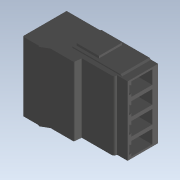
# Autodesk Inventor part: 5065752 4GD-1RR7.62-CLP-CBL
Saved by Autodesk Inventor 2021 (Build 250183000, 183)
## iProperties
Part Number: 5065752 4GD-1RR7.62-CLP-CBL
Material: Generic
Catalog Web Link: www.cadenas.de
Description: NEKM-C6 (p)-Terminal strip
Vendor: FESTO
Document SubType Name: Modeling
Designer: partserver
Manufacturer: FESTO
Mass: 15.9531 g
Surface Area: 83.8329 cm^2
Volume: 15.9531 cm^3
Density: 1 g/cm^3
Appearance: PSOLRGB-80-80-80
Categories: <MemberInstance><Categories><Category DisplayName="" Mnemonic="CABLEANDHARNESS" InternalName="e4a7e005-5e42-4d16-b293-125e7f0d0512"><Category DisplayName="" Mnemonic="CONNECTORS" InternalName="6f634eba-a678-4820-a31d-2c2d5ee6728e"><CategoryParameter DisplayName="" Mnemonic="REFDES" InternalName="c3740e8c-60ab-4d5d-8584-52b73222f2f0"/><Category DisplayName="" Mnemonic="DISCRETEWIRE" InternalName="9a3407de-09b2-4cdb-8c40-9708d5144a28"/></Category></Category></Categories><FamilyTemplate><FamilyTemplateParameters></FamilyTemplateParameters></FamilyTemplate><CategoryParameterMap><ParamToTemplateMap><ParamToTemplate CategoryParameter="//CategoryParameter[@InternalName='c3740e8c-60ab-4d5d-8584-52b73222f2f0']" ConstantValue=""/></ParamToTemplateMap></CategoryParameterMap></MemberInstance>
Category: PARTsolutions
Company: FESTO
PSOL_IDENT_0: {$CADENAS_DATA\23d-libs\festo\parts\n\nekm\parts\nekm_c6_parts.prj},199 {VTYP=3D},{NB=5065752 4GD-1R
PSOL_IDENT_1: R7.62-CLP-CBL},{LINA=5065752 4GD-1RR7.62-CLP-CBL},{NN=NEKM-C6 (p)},{DATE=16.05.2019 05:36:58},{GEOMD
PSOL_IDENT_2: ATE=16.05.2019 05:36:56},{VERSION=},{LINEID=80},{WBVAR=},{WBNUMERIC=}  {NB=5065752 4GD-1RR7.62-CLP-C
PSOL_IDENT_3: BL},{LINA=5065752 4GD-1RR7.62-CLP-CBL},{KT=DUMMY},{TNR=5065752},{TYP=4GD-1RR7.62-CLP-CBL},{VERS=5},{
PSOL_IDENT_4: N=4},{L=30.480},{L1=0.000}
NB: 5065752 4GD-1RR7.62-CLP-CBL
NN: NEKM-C6 (p)
NT: Terminal strip
NBSYN: $TNR. $TYP.
LINA: 5065752 4GD-1RR7.62-CLP-CBL
CATALOG: Festo
TNR: 5065752
TYP: 4GD-1RR7.62-CLP-CBL
VERS: 5
N: 4
L: 30.48
L1: 0
SUPPLIER: FESTO
ARTICLENO: 5065752 4GD-1RR7.62-CLP-CBL
BOMINFO: 5065752 4GD-1RR7.62-CLP-CBL
CREATOR: CADENAS GmbH
Title: 5065752 4GD-1RR7.62-CLP-CBL
Author: Cadenas PARTsolutions
Comments: Terminal strip
Autodesk Inventor part; units mm, degrees
sketch "Sketch_1" plane through (0, 0, 0) normal (0, 0, 1) x (1, 0, 0)
  line L0 (-14.7, -3.6) -> (-10.2, -3.6)
  arc A0 (-10, -3.8) -> (-10.2, -3.6) centre (-10.2, -3.8) ccw
  arc A1 (-10, -3.8) -> (-8.9, -4.9) centre (-8.9, -3.8) ccw
  line L1 (-8.9, -4.9) -> (4.3068, -4.9)
  line L2 (4.3068, -4.9) -> (4.5468, -7.6436)
  arc A2 (4.5468, -7.6436) -> (5.0449, -8.1) centre (5.0449, -7.6) ccw
  line L3 (5.0449, -8.1) -> (14.9, -8.1)
  line L4 (14.9, -8.1) -> (18.0177, -9.9)
  line L5 (18.0177, -9.9) -> (18.3, -9.9)
  arc A3 (18.3, -9.9) -> (18.5, -9.7) centre (18.3, -9.7) ccw
  line L6 (18.5, -9.7) -> (18.5, -9.6)
  line L7 (18.5, -9.6) -> (25.3, -9.6)
  arc A4 (25.3, -9.6) -> (25.8, -9.1) centre (25.3, -9.1) ccw
  line L8 (25.8, -9.1) -> (25.8, 9.9)
  line L9 (25.8, 9.9) -> (-14.7, 9.9)
  line L10 (-14.7, 9.9) -> (-14.7, -3.6)
  constraints: 22 end point, 10 point on circle, 5 centre point
extrude "Extrusion1" add sketch "Sketch_1" along normal mid plane 30.48
sketch "Sketch_2" plane through (0, 9.9, 0) normal (0, 1, 0) x (1, 0, 0)
  line L0 (-11.6, 15.24) -> (-11.6, -15.24)
  line L1 (-11.6, -15.24) -> (-10.8206, -15.69)
  line L2 (-10.8206, -15.69) -> (10.45, -15.69)
  line L3 (10.45, -15.69) -> (10.45, 15.69)
  line L4 (10.45, 15.69) -> (-10.8206, 15.69)
  line L5 (-10.8206, 15.69) -> (-11.6, 15.24)
  constraints: 12 end point
extrude "Extrusion2" add sketch "Sketch_2" against normal blind 12.825
sketch "Sketch_3" plane through (0, 0, 0) normal (0, 0, 1) x (1, 0, 0)
  line L0 (0, -1.625) -> (9.8, -1.625)
  line L1 (9.8, -1.625) -> (9.8, 8.575)
  line L2 (9.8, 8.575) -> (0, 8.575)
  line L3 (0, 8.575) -> (0, -1.625)
  constraints: 8 end point
extrude "Extrusion3" add sketch "Sketch_3" along normal mid plane 33.28
sketch "Sketch_4" plane through (26.75, 0, 0) normal (1, 0, 0) x (0, 0, -1)
  line L0 (-14.64, 6.0143) -> (-14.64, 3.1857)
  arc A0 (-14.64, 3.1857) -> (-8.22, 3.1857) centre (-11.43, 4.45) ccw
  line L1 (-8.22, 3.1857) -> (-8.22, 6.0143)
  arc A1 (-8.22, 6.0143) -> (-14.64, 6.0143) centre (-11.43, 4.75) ccw
  constraints: 4 end point, 4 point on circle, 2 centre point
extrude "Extrusion4" cut sketch "Sketch_4" against normal blind 10
pattern_linear "Rectangular Pattern1" count 4 spacing 7.62 along (0, 0, -1) of "Extrusion4"
sketch "Sketch_6" plane through (26.75, 0, 0) normal (1, 0, 0) x (0, 0, -1)
  line L0 (-13.28, -4.05) -> (-9.58, -4.05)
  line L1 (-9.58, -4.05) -> (-9.58, -0.2)
  line L2 (-9.58, -0.2) -> (-13.28, -0.2)
  line L3 (-13.28, -0.2) -> (-13.28, -4.05)
  constraints: 8 end point
extrude "Extrusion5" cut sketch "Sketch_6" against normal blind 7
pattern_linear "Rectangular Pattern2" count 4 spacing 7.62 along (0, 0, -1) of "Extrusion5"
sketch "Sketch_8" plane through (-14.7, 0, 0) normal (1, 0, 0) x (0, 0, -1)
  line L0 (-14.41, -1.925) -> (-13.1415, -1.925)
  arc A0 (-12.9485, -2.1178) -> (-13.1415, -1.925) centre (-13.1415, -2.118) ccw
  arc A1 (-13.0174, -2.2655) -> (-12.9485, -2.1178) centre (-13.1415, -2.1177) ccw
  line L1 (-13.0174, -2.2655) -> (-13.302, -2.5043)
  arc A2 (-13.302, -2.5043) -> (-13.1776, -2.846) centre (-13.1776, -2.6525) ccw
  line L2 (-13.1776, -2.846) -> (-9.6824, -2.846)
  arc A3 (-9.6824, -2.846) -> (-9.558, -2.5043) centre (-9.6824, -2.6525) ccw
  line L3 (-9.558, -2.5043) -> (-9.8426, -2.2655)
  arc A4 (-9.9115, -2.1178) -> (-9.8426, -2.2655) centre (-9.7185, -2.1177) ccw
  arc A5 (-9.7185, -1.925) -> (-9.9115, -2.1178) centre (-9.7185, -2.118) ccw
  line L4 (-9.7185, -1.925) -> (-8.45, -1.925)
  line L5 (-8.45, -1.925) -> (-8.45, 7.325)
  line L6 (-8.45, 7.325) -> (-14.41, 7.325)
  line L7 (-14.41, 7.325) -> (-14.41, -1.925)
  constraints: 16 end point, 12 point on circle, 6 centre point
extrude "Extrusion6" cut sketch "Sketch_8" along normal blind 14.7
pattern_linear "Rectangular Pattern3" count 4 spacing 7.62 along (0, 0, -1) of "Extrusion6"
sketch "Sketch_10" plane through (0, 0, 0) normal (1, 0, 0) x (0, 1, 0)
  circle A0 centre (3.475, 11.43) radius 1.6
  constraints: 1 centre point
extrude "Extrusion7" add sketch "Sketch_10" against normal blind 1
pattern_linear "Rectangular Pattern4" count 4 spacing 7.62 along (0, 0, -1) of "Extrusion7"
sketch "Sketch_12" plane through (0, 0, 0) normal (1, 0, 0) x (0, 1, 0)
  line L0 (3.075, 12.93) -> (3.075, 9.93)
  line L1 (3.075, 9.93) -> (3.875, 9.93)
  line L2 (3.875, 9.93) -> (3.875, 12.93)
  line L3 (3.875, 12.93) -> (3.075, 12.93)
  constraints: 8 end point
extrude "Extrusion8" add sketch "Sketch_12" against normal blind 5.95
pattern_linear "Rectangular Pattern5" count 4 spacing 7.62 along (0, 0, -1) of "Extrusion8"
ref_plane "ANBAU_XY" through (0, 0, 0) normal (0, 1, 0) x (1, 0, 0)
ref_plane "ANBAU_YZ" through (0, 0, 0) normal (1, 0, 0) x (0, 0, -1)
ref_plane "ANBAU_ZX" through (0, 0, 0) normal (0, 0, -1) x (0, 1, 0)
sketch "Sketch9" plane through (25.8, -9.1, 15.24) normal (1, 0, 0) x (0, 0, -1)
  arc A0 (23.46, 12.2857) -> (29.88, 12.2857) centre (26.67, 13.55) ccw projected
sketch "Sketch10" plane through (25.8, -9.1, 15.24) normal (1, 0, 0) x (0, 0, -1)
  arc A0 (15.84, 12.2857) -> (22.26, 12.2857) centre (19.05, 13.55) ccw projected
sketch "Sketch11" plane through (25.8, -9.1, 15.24) normal (1, 0, 0) x (0, 0, -1)
  arc A0 (8.22, 12.2857) -> (14.64, 12.2857) centre (11.43, 13.55) ccw projected
sketch "Sketch12" plane through (25.8, -9.1, 15.24) normal (1, 0, 0) x (0, 0, -1)
  arc A0 (0.6, 12.2857) -> (7.02, 12.2857) centre (3.81, 13.55) ccw projected
body "Solid1"
